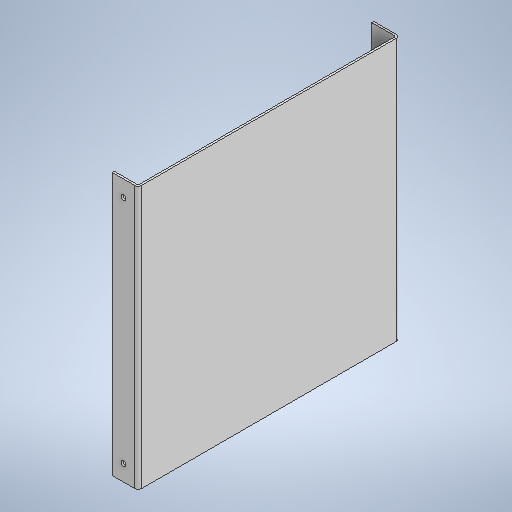
# Autodesk Inventor part: fire wall
Saved by Autodesk Inventor 2025.2 (Build 292293000, 293)
## iProperties
Created: 2025-02-04
Part Number: fire wall
Material: Generic
Document SubType Name: Sheet Metal
Designer: 5013908
Density: 1 g/cm^3
Sheet Metal Rule: Default
Appearance: Default
Author: 5013908
Autodesk Inventor part; units mm, degrees
ref_plane "YZ Plane" through (0, 0, 0) normal (1, 0, 0) x (0, 1, 0)
ref_plane "XZ Plane" through (0, 0, 0) normal (0, 1, 0) x (-1, 0, 0)
ref_plane "XY Plane" through (0, 0, 0) normal (0, 0, 1) x (1, 0, 0)
sketch "Sketch1" plane through (0, 0, 0) normal (0, 1, 0) x (-1, 0, 0)
  line L0 (0, -2) -> (0, -403)
  line L1 (2, -405) -> (40, -405)
  line L2 (40, -405) -> (40, -401.825)
  line L3 (40, -401.825) -> (5.175, -401.825)
  line L4 (3.175, -399.825) -> (3.175, -5.175)
  line L5 (5.175, -3.175) -> (40, -3.175)
  line L6 (40, -3.175) -> (40, 0)
  line L7 (40, 0) -> (2, 0)
  arc A0 (5.175, -3.175) -> (3.175, -5.175) centre (5.175, -5.175) ccw
  arc A1 (3.175, -399.825) -> (5.175, -401.825) centre (5.175, -399.825) ccw
  arc A2 (0, -403) -> (2, -405) centre (2, -403) ccw
  arc A3 (5.175, 0) -> (0, -5.175) centre (5.175, -5.175) ccw
  arc A4 (0, -399.825) -> (5.175, -405) centre (5.175, -399.825) ccw
  point P0 (0, 0)
  point P1 (0, -405)
  dimension "d0" = 405
  dimension "d1" = 40
  dimension "d2" = 3.175
  dimension "d3" = 3.175
  dimension "d4" = 3.175
  dimension "d5" = 40
  dimension "d6" = 2
  constraints: 16 end point, 10 point on circle, 8 point on line, 6 perpendicular, 6 tangent, 5 centre point, 2 coincident, 2 equal radius, 1 parallel, 1 vertical
  measures "d0" distance of point (0, 0) point (0, -405)
  measures "d1" distance of point (0, -405) L1.end
  measures "d2" distance of L1.end L2.end
  measures "d3" distance of L5.end L6.end
  measures "d4" distance between parallel lines of L0 L4
  measures "d5" distance of L6.end point (0, 0)
  measures "d6" radius of A0
extrude "Extrusion1" add sketch "Sketch1" along normal blind 406.5 contours A3 L7 L6 L5 A0 L4 A1 L3 L2 L1 A4 L0
sketch "Sketch2" plane through (-2, 0, -405) normal (0, 0, -1) x (-1, 0, 0)
  circle A0 centre (20.5875, 25) radius 4
  circle A1 centre (20.5875, 381.5) radius 4
  line L0 (3.175, 406.5) -> (38, 406.5) projected
  line L1 (3.175, 0) -> (38, 0) projected
  line L2 (38, 0) -> (38, 406.5) projected
  line L3 (3.175, 0) -> (3.175, 406.5) projected
  point P0 (-2, 0)
  point P1 (0, 406.5)
  point P2 (20.5875, 406.5)
  point P3 (0, 0)
  point P4 (20.5875, 406.5)
  point P5 (20.5875, 0)
  dimension "d9" = 8
  dimension "d10" = 8
  dimension "d11" = 25
  dimension "d12" = 25
  dimension "d19" = 0
  dimension "d20" = 0
  constraints: 3 midpoint, 2 centre point
  measures "d9" diameter of A0
  measures "d10" diameter of A1
  measures "d11" distance of point (20.588, 406.5) A1.centre
  measures "d12" distance from line of L1 A0.centre
  measures "d19" horizontal distance of point (20.588, 406.5) A1.centre
  measures "d20" horizontal distance of point (20.588, 0) A0.centre
extrude "Extrusion2" cut sketch "Sketch2" against normal blind 451.5 contours A0 | A1
equation "\"BendRadius\" = Thickness"
equation "\"BendReliefWidth\" = Thickness"
equation "\"BendReliefDepth\" = 0.5 * Thickness"
equation "\"CornerReliefSize\" = 4 * Thickness"
equation "\"MinimumRemnant\" = 2 * Thickness"
equation "\"TransitionRadius\" = BendRadius"
equation "\"JacobiRadiusSize\" = BendRadius"
equation "\"GapSize\" = Thickness"
equation "\"Thickness\" = 3.048"
body "Solid1"
